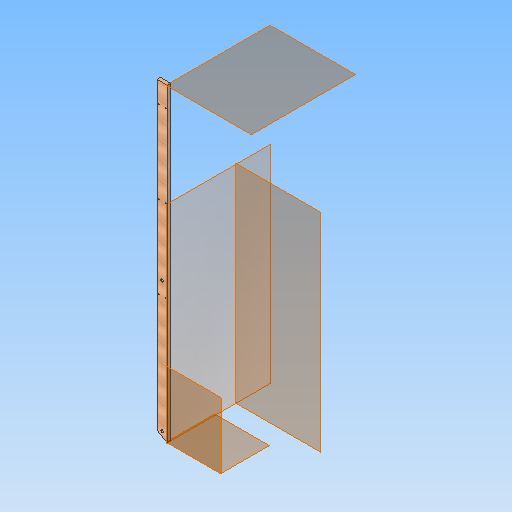
# Autodesk Inventor part: Top_Reinforcement_LHS
Saved by Autodesk Inventor 2018.1 (Build 221171000, 171)
## iProperties
Created: 2019-03-15
Part Number: Top_Reinforcement_LHS
Material: Wood (Birch)
Document SubType Name: Modeling
Designer: James
Density: 0.55 g/cm^3
Appearance: Birch - Natural Polished
Author: James
Autodesk Inventor part; units mm, degrees
ref_plane "YZ Plane" through (0, 0, 0) normal (1, 0, 0) x (0, 1, 0)
ref_plane "XZ Plane" through (0, 0, 0) normal (0, 1, 0) x (-1, 0, 0)
ref_plane "XY Plane" through (0, 0, 0) normal (0, 0, 1) x (1, 0, 0)
derived "Top_Skeleton.ipt"
ref_plane "Work Plane1" through (0, 0, 0) normal (0, 0, 1) x (1, 0, 0)
ref_plane "Work Plane2" through (0, 0, 0) normal (0, 1, 0) x (-1, 0, 0)
ref_plane "Work Plane3" through (0, 0, 0) normal (1, 0, 0) x (0, 1, 0)
ref_plane "Work Plane4" through (0, 4500, 0) normal (0, 1, 0) x (-1, 0, 0)
ref_plane "Work Plane5" through (0, 0, -1000) normal (0, 0, 1) x (1, 0, 0)
sketch "Sketch1" plane through (0, 0, 0) normal (1, 0, 0) x (0, 1, 0)
  line L0 (0, 0) -> (4500, 0)
  line L1 (4500, 0) -> (4500, -50)
  line L2 (4500, -50) -> (0, -50)
  line L3 (0, -50) -> (0, 0)
  line L4 (4500, 10) -> (4500, -60) projected
  dimension "d1" = 50
  constraints: 8 end point, 2 parallel, 1 coincident, 1 horizontal, 1 perpendicular, 1 point on line
  measures "d1" distance of L0.end L1.end
extrude "Extrusion1" add sketch "Sketch1" against normal blind 150
chamfer "Chamfer1" distance 130 angle 30 1 edges at (-150, 0, -25) measured on face at (-149.5, 0, -25)
sketch "Sketch2" plane through (0, 0, 0) normal (0, 0, 1) x (1, 0, 0)
  line L0 (-150, 75.0555) -> (-150, 4500) projected
  line L1 (0, 5400) -> (0, -900) projected
  line L2 (0, 0) -> (-20, 0) projected
  point P0 (-75, 100)
  point P1 (-75, 2000)
  dimension "d7" = 75
  dimension "d8" = 75
  dimension "d9" = 100
  dimension "d33" = 2000
  constraints: 1 vertical alignment
  measures "d7" distance from line of L0 point (-75, 100)
  measures "d8" distance from line of L1 point (-75, 100)
  measures "d9" distance from line of L2 point (-75, 100)
  measures "d33" distance from line of L2 point (-75, 2000)
hole "Hole1" at (-75, 100, 0) at (-75, 2000, 0) direction (0, 0, -1) diameter 30 end through all
chamfer "Chamfer2" distance 5 angle 45 4 edges at (-75, 115, -50) (-75, 115, 0) (-75, 2015, -50) (-75, 2015, 0)
sketch "Sketch3" plane through (0, 0, 0) normal (0, 0, 1) x (1, 0, 0)
  line L0 (-150, 75.0555) -> (-150, 4500) projected
  line L1 (0, 5400) -> (0, -900) projected
  line L2 (0, 4500) -> (-150, 4500) projected
  point P0 (0, 0)
  point P1 (-125, 4200)
  point P2 (-25, 4200)
  dimension "d20" = 25
  dimension "d21" = 25
  dimension "d22" = 300
  constraints: 1 horizontal alignment
  measures "d20" distance from line of L0 point (-125, 4200)
  measures "d21" distance from line of L1 point (-25, 4200)
  measures "d22" distance from line of L2 point (-125, 4200)
hole "Hole2" at (-125, 4200, 0) at (-25, 4200, 0) direction (0, 0, -1) diameter 8.433 end through all countersink diameter 16.129 countersink angle 82 clearance for "Flat Head Machine Screw (82)" size "5/16" standard "Ansi Unified Screw Threads"
pattern_linear "Rectangular Pattern1" count 3 spacing 1200 along (0, -1, 0) of "Hole2"
sketch "Sketch4" plane through (0, 0, -50) normal (0, 0, -1) x (-1, 0, 0)
  circle A0 centre (75, 2000) radius 20 projected
  point P0 (0, 0)
  point P1 (25, 1950)
  point P2 (25, 2050)
  point P3 (125, 2050)
  point P4 (125, 1950)
  dimension "d34" = 50
  dimension "d35" = 100
  dimension "d36" = 100
  dimension "d37" = 50
  constraints: 2 horizontal alignment, 2 vertical alignment
  measures "d34" horizontal distance of A0.centre point (25, 2050)
  measures "d35" distance of point (25, 2050) point (125, 2050)
  measures "d36" distance of point (125, 1950) point (125, 2050)
  measures "d37" horizontal distance of A0.centre point (125, 2050)
hole "Hole3" at (-25, 1950, -50) at (-25, 2050, -50) at (-125, 2050, -50) at (-125, 1950, -50) direction (0, 0, 1) diameter 6.401 depth 22.931 tip angle 118 thread size "5/16-18 UNC" class "2B" standard "ANSI Unified Screw Threads"
equation "\"d7\" = d8"
equation "\"d21\" = d20"
equation "\"d34\" = 0.5 * d35"
equation "\"d36\" = d35"
equation "\"d37\" = 0.5 * d36"
body "Solid1"
